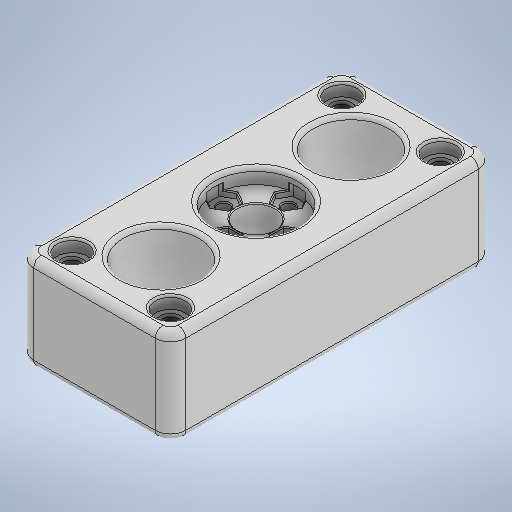
# Autodesk Inventor part: guia superior
Saved by Autodesk Inventor 2025.2 (Build 292293000, 293)
## iProperties
Created: 2025-10-16
Part Number: guia superior
Material: Genérico
Document SubType Name: Modeling
Designer: Jonathan Galarza
Density: 1 g/cm^3
Appearance: Valor por defecto
Author: Jonathan Galarza
Autodesk Inventor part; units mm, degrees
ref_plane "YZ Plane" through (0, 0, 0) normal (1, 0, 0) x (0, 1, 0)
ref_plane "XZ Plane" through (0, 0, 0) normal (0, 1, 0) x (-1, 0, 0)
ref_plane "XY Plane" through (0, 0, 0) normal (0, 0, 1) x (1, 0, 0)
sketch "Boceto1" plane through (0, 0, 0) normal (0, 1, 0) x (-1, 0, 0)
  line L0 (-20, -42.5) -> (20, -42.5)
  line L1 (20, -42.5) -> (20, 42.5)
  line L2 (20, 42.5) -> (-20, 42.5)
  line L3 (-20, 42.5) -> (-20, -42.5)
  line L4 (-20, -42.5) -> (20, 42.5) construction
  line L5 (20, -42.5) -> (-20, 42.5) construction
  line L6 (15.6711, 0) -> (-15.6711, 0) construction
  line L7 (0, 25) -> (0, -25) construction
  circle A0 centre (0, 25) radius 7.5
  circle A1 centre (0, -25) radius 7.5
  circle A2 centre (0, 25) radius 10
  circle A3 centre (0, -25) radius 10
  circle A4 centre (-13, -35.5) radius 2.25
  line L8 (15.6711, 0) -> (-15.6711, 0)
  line L9 (0, -12.7103) -> (0, 13.5129)
  circle A5 centre (-13, 35.5) radius 2.25
  circle A6 centre (13, -35.5) radius 2.25
  circle A7 centre (13, 35.5) radius 2.25
  point P0 (0, 0)
  point P1 (0, 35)
  point P2 (0, -35)
  dimension "d0" = 40
  dimension "d1" = 85
  dimension "d3" = 50
  dimension "d6" = 15
  dimension "d7" = 15
  dimension "d27" = 4.5
  dimension "d28" = 7
  dimension "d29" = 7
  constraints: 20 end point, 8 centre point, 4 coincident, 4 midpoint, 3 horizontal, 3 symmetric about line, 2 parallel, 2 point on line, 1 perpendicular, 1 vertical, 3 other
  measures "d0" distance of L2.end L1.end
  measures "d1" distance of L1.end L0.end
  measures "d3" distance of L7.start L7.end
  measures "d6" diameter of A0
  measures "d7" diameter of A1
  measures "d27" diameter of A4
  measures "d28" distance from line of L3 A4.centre
  measures "d29" distance from line of L0 A4.centre
extrude "Extrusión1" add sketch "Boceto1" along normal blind 25 contours L3 L2 L1 L0
fillet "Empalme1" radius 4 4 edges at (20, 12.5, -42.5) (20, 12.5, 42.5) (-20, 12.5, 42.5) (-20, 12.5, -42.5)
fillet "Empalme2" radius 2 16 edges at (-18.8284, 25, 41.3284) (0, 25, 42.5) (18.8284, 25, 41.3284) (20, 25, 0) (18.8284, 25, -41.3284) (0, 25, -42.5) (-18.8284, 25, -41.3284) (-20, 25, 0) (-18.8284, 0, 41.3284) (0, 0, 42.5) (18.8284, 0, 41.3284) (20, 0, 0) (18.8284, 0, -41.3284) (0, 0, -42.5) (-18.8284, 0, -41.3284) (-20, 0, 0)
sketch "Boceto3" plane through (0, 25, 0) normal (0, 1, 0) x (1, 0, 0)
  circle A0 centre (13, 35.5) radius 2.25 projected
  circle A1 centre (13, 35.5) radius 4
  line L0 (-7.5192, 0) -> (7.6222, 0)
  line L1 (0.0515, -5.5954) -> (0.0515, 7.1321)
  circle A2 centre (13, -35.5) radius 4
  circle A3 centre (-12.897, 35.5) radius 4
  circle A4 centre (-12.897, -35.5) radius 4
  point P0 (0, 0)
  dimension "d30" = 8
  constraints: 4 centre point, 4 end point, 3 symmetric about line, 1 coincident, 1 horizontal, 1 vertical, 3 other
  measures "d30" diameter of A1
extrude "Extrusión4" cut sketch "Boceto3" against normal blind 3.25 contours A0 | A1 | A2 | A3 | A4
fillet "Empalme3" radius 0.5 4 edges at (-16.897, 25, 35.5) (9, 25, 35.5) (9, 25, -35.5) (-16.897, 25, -35.5)
fillet "Empalme4" radius 0.5 8 edges at (-10.75, 21.75, -35.5) (15.25, 21.75, -35.5) (-10.75, 21.75, 35.5) (15.25, 21.75, 35.5) (15.25, 0, 35.5) (-10.75, 0, 35.5) (15.25, 0, -35.5) (-10.75, 0, -35.5)
sketch "Boceto4" plane through (0, 25, 0) normal (0, 1, 0) x (1, 0, 0)
  circle A0 centre (0, 0) radius 5
  dimension "d35" = 10
  constraints: 1 centre point, 1 coincident
  measures "d35" diameter of A0
extrude "Extrusión5" cut sketch "Boceto4" against normal through all
sketch "Boceto5" plane through (0, 25, 0) normal (0, 1, 0) x (1, 0, 0)
  circle A0 centre (0, 0) radius 11
  dimension "d38" = 22
  constraints: 1 centre point, 1 coincident
  measures "d38" diameter of A0
extrude "Extrusión6" cut sketch "Boceto5" against normal blind 4
sketch "Boceto6" plane through (0, 21, 0) normal (0, 1, 0) x (1, 0, 0)
  circle A0 centre (0, 0) radius 11 projected
  line L0 (0, 11) -> (0, 10)
  circle A1 centre (0, 8.5) radius 1.5
  circle A2 centre (-8.5, 0) radius 1.5
  circle A3 centre (0, -8.5) radius 1.5
  circle A4 centre (8.5, 0) radius 1.5
  dimension "d41" = 1
  dimension "d42" = 3
  dimension "d43" = 1
  dimension "d46" = 360
  constraints: 4 centre point, 2 end point, 1 vertical, 1 vertical alignment, 10 other
  measures "d41" distance of L0.start L0.end
  measures "d42" diameter of A1
extrude "Extrusión7" cut sketch "Boceto6" against normal through all contours A1 | A2 | A3 | A4
sketch "Boceto7" plane through (0, 21, 0) normal (0, 1, 0) x (1, 0, 0)
  circle A0 centre (0, 8.5) radius 1.5 projected
  line L0 (-1.7321, 5.5) -> (-3.4641, 8.5)
  line L1 (-3.4641, 8.5) -> (-1.7321, 11.5)
  line L2 (-1.7321, 11.5) -> (1.7321, 11.5)
  line L3 (1.7321, 11.5) -> (3.4641, 8.5)
  line L4 (3.4641, 8.5) -> (1.7321, 5.5)
  line L5 (1.7321, 5.5) -> (-1.7321, 5.5)
  line L6 (-8.5, 3.4641) -> (-5.5, 1.7321)
  line L7 (-11.5, 1.7321) -> (-8.5, 3.4641)
  line L8 (-11.5, -1.7321) -> (-11.5, 1.7321)
  line L9 (-8.5, -3.4641) -> (-11.5, -1.7321)
  line L10 (-5.5, -1.7321) -> (-8.5, -3.4641)
  line L11 (-5.5, 1.7321) -> (-5.5, -1.7321)
  line L12 (-3.4641, -8.5) -> (-1.7321, -5.5)
  line L13 (-1.7321, -11.5) -> (-3.4641, -8.5)
  line L14 (1.7321, -11.5) -> (-1.7321, -11.5)
  line L15 (3.4641, -8.5) -> (1.7321, -11.5)
  line L16 (1.7321, -5.5) -> (3.4641, -8.5)
  line L17 (-1.7321, -5.5) -> (1.7321, -5.5)
  line L18 (8.5, -3.4641) -> (5.5, -1.7321)
  line L19 (11.5, -1.7321) -> (8.5, -3.4641)
  line L20 (11.5, 1.7321) -> (11.5, -1.7321)
  line L21 (8.5, 3.4641) -> (11.5, 1.7321)
  line L22 (5.5, 1.7321) -> (8.5, 3.4641)
  line L23 (5.5, -1.7321) -> (5.5, 1.7321)
  point P0 (0, 0)
  dimension "d50" = 6
  dimension "d53" = 360
  constraints: 48 end point, 1 coincident, 62 other
  measures "d50" distance between parallel lines of L5 L2
extrude "Extrusión8" cut sketch "Boceto7" along normal mid plane 3 contours A0 | L0 L1 L2 L3 L4 L5 | L6 L11 L10 L9 L8 L7 | L12 L17 L16 L15 L14 L13 | L18 L23 L22 L21 L20 L19
fillet "Empalme5" radius 1 5 edges at (-11, 25, 0) (10, 25, -25) (10, 25, 25) (10, 0, 25) (10, 0, -25)
fillet "Empalme6" radius 0.25 43 edges at (-5, 0, 0) (-5, 21, 0) (-5.5, 21, 0) (-7, 21, -2.5981) (-9.6447, 21, -2.8032) (-9.6447, 21, 2.8032) (-7, 21, 2.5981) (-2.8032, 21, -9.6447) (-2.5981, 21, -7) (2.5981, 21, -7) (2.8032, 21, -9.6447) (0, 21, -5.5) (-1.5, 19.5, -8.5) (-10, 19.5, 0) (7, 21, 2.5981) (9.6447, 21, 2.8032) (7, 19.5, 0) (9.6447, 21, -2.8032) (7, 21, -2.5981) (5.5, 21, 0) (2.8032, 21, 9.6447) (2.5981, 21, 7) (0, 21, 5.5) (-2.5981, 21, 7) (-2.8032, 21, 9.6447) (-1.5, 19.5, 8.5) (-2.1423, 21.75, -10.7894) (0, 22.5, -11) (2.1423, 21.75, -10.7894) (-11, 22.5, 0) (-10.7894, 21.75, -2.1423) (-10.7894, 21.75, 2.1423) (10.9472, 22.5, 1.0763) (10.9472, 22.5, -1.0763) (10.7894, 21.75, 2.1423) (10.7894, 21.75, -2.1423) (0, 22.5, 11) (-2.1423, 21.75, 10.7894) (2.1423, 21.75, 10.7894) (-1.5, 0, 8.5) (7, 0, 0) (-10, 0, 0) (-1.5, 0, -8.5)
